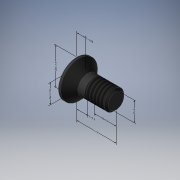
# Autodesk Inventor part: Senkschraube DIN ≈965 M4x8 51305.040.008(High)
Saved by Autodesk Inventor 2019 (Build 230136000, 136)
## iProperties
Created: 2022-09-09
Part Number: Senkschraube DIN ≈965 M4x8 51305.040.008(High)
Material: Generic
Catalog Web Link: www.cadenas.de
Description: DIN ≈965-Counter sunk screws with torx
Vendor: FABORY
Document SubType Name: Modeling
Designer: psAdmin
Manufacturer: FABORY
Mass: 1 g
Surface Area: 2.10234 cm^2
Volume: 0.118629 cm^3
Density: 1 g/cm^3
Appearance: PSOLRGB-175-175-175
Category: PARTsolutions
Company: FABORY
Title: Senkschraube DIN ≈965 M4x8
Author: Cadenas PARTsolutions
Comments: Counter sunk screws with torx
PSOL_IDENT_0: {$CADENAS_DATA/23d-libs/fabory/6_screws/din_965_v2.prj},220 {VTYP=3D},{NB=Senkschraube DIN ≈965 M4x8
PSOL_IDENT_1: 51305.040.008(High)},{LINA=Senkschraube DIN ≈965 M4x8},{NN=DIN ≈965},{DATE=02.05.2022 11:12:59},{GE
PSOL_IDENT_2: OMDATE=13.03.2019 09:47:59},{VERSION=},{LINEID=54070},{WBVAR=LOD},{WBNUMERIC=}  {NB=Senkschraube DIN
PSOL_IDENT_3: ≈965 M4x8 51305.040.008(High)},{LINA=Senkschraube DIN ≈965 M4x8},{KT=DUMMY},{CNSORDERNO=51305.040.0
PSOL_IDENT_4: 08},{NENNID=M4x8},{D=4.000},{L=8},{ERPPDMNUMBER=51305.040.008},{BRAND=Fabory},{STANDARD=DIN ≈965},{T
PSOL_IDENT_5: HREAD=Metric thread},{THREADDIRECTION=},{STYLE=},{TYPE=Machine screw},{GRADE=A2},{BASICMATERIAL=Stai
PSOL_IDENT_6: nless steel},{SURFACETREATMEN=},{HEADSHAPE=Countersunk head},{DRIVINGFEATURE=Hexalobular},{CNSMASSEX
PSOL_IDENT_7: ACT=0.0009},{COLOR=},{COMPARABLESTAND=ISO≈14581;NF≈E25-119-1},{ADDITIONALINFO=Metric},{ROHS=Y},{APPR
PSOL_IDENT_8: OVAL=},{EANCODE=8715494160254},{INTRASTCODE=},{ECLASS=},{UNSPSC=31161504},{ETIM=EC000887},{URL=https
PSOL_IDENT_9: ://www.fabory.com/en-GB/p/51305040008},{PACKAGING=MIN},{VARIANT=MIN},{FABNENN=},{FABGEO=},{FABARTICL
PSOL_IDENT_10: ENR=51305.040.008},{FABNETWEIGHT=0.900},{NENN=M4x8},{D3=3.141},{P=0.700},{DIN962THREAD=},{XLH=0},{DI
PSOL_IDENT_11: N962OPT2=},{OPTIONS2L='',' - ','din_962_std_mid.jpg'},{DIN962OPT3=},{OPTIONSS='',' - ','din_962_std_
PSOL_IDENT_12: gew.jpg'},{B=4.400},{B2=22.000},{A1=1.400},{DK=7.50},{K=2.200},{R=0.400},{X=1.25},{NR=20},{A=3.95},{
PSOL_IDENT_13: T=1.66},{NRP=MIN},{M=MIN},{SCLN=3.5},{SCDN=2.88},{SCLK=2.1},{Z0H=0.8},{Z0D2=8},{Z1H=0.8},{Z1D2=9},{Z
PSOL_IDENT_14: 2H=1},{Z2D2=12},{SD1=1},{SLE=2.2},{FLDP=2.5},{CPDZ=2},{TCDT=0},{SDDP=2.5},{SDZ1=1},{LDDP=2.5},{LDZ2=
PSOL_IDENT_15: 2},{DIN962FTHREAD=0},{VERS=1},{CNSAVOID=0},{DIST=0.31},{LINK1=51305},{LINK2=040},{LINK3=008},{INFOPA
PSOL_IDENT_16: TH=https://www.fabory.com/en-GB/p/51305040008},{LOD=High},{STANDARDSMALL=din_965_v2.png}
NB: Senkschraube DIN ≈965 M4x8 51305.040.008(High)
NN: DIN ≈965
NT: Counter sunk screws with torx
NBSYN: Senkschraube DIN ≈965 $NENN. $CNSORDERNO.($LOD.)
LINA: Senkschraube DIN ≈965 M4x8
CATALOG: Fabory
ROWDESC: M4x8
OFFICIAL_STANDARD_NUMBERS: ISO 14581
CNSORDERNO: 51305.040.008
NENNID: M4x8
D: 4
L: 8
BRAND: Fabory
STANDARD: DIN ≈965
THREAD: Metric thread
TYPE: Machine screw
GRADE: A2
BASICMATERIAL: Stainless steel
HEADSHAPE: Countersunk head
DRIVINGFEATURE: Hexalobular
CNSMASSEXACT: 0.001
COMPARABLESTAND: ISO≈14581;NF≈E25-119-1
ROHS: Y
EANCODE: 8715494160254
UNSPSC: 31161504
ETIM: EC000887
URL: https://www.fabory.com/en-GB/p/51305040008
D3: 3.141
P: 0.7
B: 4.4
B2: 22
A1: 1.4
DK: 7.5
K: 2.2
R: 0.4
X: 1.25
NR: 20
A: 3.95
T: 1.66
NRP: 0
M: 0
SUPPLIER: FABORY
ARTICLENO: Senkschraube DIN ≈965 M4x8 51305.040.008(High)
BOMINFO: Senkschraube DIN ≈965 M4x8
CREATOR: CADENAS GmbH
Autodesk Inventor part; units mm, degrees
sketch "Skizze_5" plane through (0, 0, 0) normal (0, 0, 1) x (1, 0, 0)
  line L0 (8, 0) -> (0, 0)
  line L1 (0, 0) -> (0, 3.75)
  line L2 (0, 3.75) -> (0.45, 3.75)
  line L3 (0.45, 3.75) -> (2.2, 2)
  line L4 (2.2, 2) -> (7.5705, 2)
  line L5 (7.5705, 2) -> (8, 1.5705)
  line L6 (8, 1.5705) -> (8, 0)
  line L7 (8, 0) -> (0, 0)
  constraints: 16 end point
revolve "Revolution1" add sketch "Skizze_5" angle 360 about axis through (8, 0, 0) along (1, 0, 0)
thread "Thread1" size "M4x0.7" class "6g" standard "ISO Metric profile" length 3.9705
sketch "Sketch_1" plane through (0, 0, 0) normal (0, 0, 1) x (1, 0, 0)
  line L0 (1.66, 0) -> (0, 0)
  line L1 (0, 0) -> (0, 1.975)
  line L2 (0, 1.975) -> (1.66, 1.975)
  line L3 (1.66, 1.975) -> (1.66, 0)
  line L4 (1.66, 0) -> (0, 0)
  constraints: 10 end point
revolve "Revolution2" cut sketch "Sketch_1" angle 360 about axis through (1.66, 0, 0) along (1, 0, 0)
sketch "Sketch_2" plane through (0, 0, 0) normal (0, 0, 1) x (1, 0, 0)
  line L0 (2.8003, 0) -> (1.66, 0)
  line L1 (1.66, 0) -> (1.66, 1.975)
  line L2 (1.66, 1.975) -> (2.8003, 0)
  line L3 (2.8003, 0) -> (1.66, 0)
  constraints: 8 end point
revolve "Revolution3" cut sketch "Sketch_2" angle 360 about axis through (2.8003, 0, 0) along (1, 0, 0)
sketch "Sketch_3" plane through (0, 0, 0) normal (1, 0, 0) x (0, 1, 0)
  circle A0 centre (0, 0) radius 2.37
  arc A1 (-0.5027, 1.6394) -> (-1.1684, 1.2551) centre (-0.79, 1.3683) ccw
  arc A2 (-1.6711, 0.3843) -> (-1.1684, 1.2551) centre (-1.8307, 1.0569) ccw
  arc A3 (-1.6711, 0.3843) -> (-1.6711, -0.3843) centre (-1.58, 0) ccw
  arc A4 (-1.1684, -1.2551) -> (-1.6711, -0.3843) centre (-1.8307, -1.0569) ccw
  arc A5 (-1.1684, -1.2551) -> (-0.5027, -1.6394) centre (-0.79, -1.3683) ccw
  arc A6 (0.5027, -1.6394) -> (-0.5027, -1.6394) centre (0, -2.1139) ccw
  arc A7 (0.5027, -1.6394) -> (1.1684, -1.2551) centre (0.79, -1.3683) ccw
  arc A8 (1.6711, -0.3843) -> (1.1684, -1.2551) centre (1.8307, -1.0569) ccw
  arc A9 (1.6711, -0.3843) -> (1.6711, 0.3843) centre (1.58, 0) ccw
  arc A10 (1.1684, 1.2551) -> (1.6711, 0.3843) centre (1.8307, 1.0569) ccw
  arc A11 (1.1684, 1.2551) -> (0.5027, 1.6394) centre (0.79, 1.3683) ccw
  arc A12 (-0.5027, 1.6394) -> (0.5027, 1.6394) centre (0, 2.1139) ccw
  constraints: 24 point on circle, 13 centre point
extrude "Extrusion1" add sketch "Sketch_3" along normal blind 1.66
sketch "Sketch_4" plane through (0, 0, 0) normal (0, 0, 1) x (1, 0, 0)
  line L0 (1.1403, 0) -> (-1.66, 0)
  line L1 (-1.66, 0) -> (-1.66, 1.975)
  line L2 (-1.66, 1.975) -> (0, 1.975)
  line L3 (0, 1.975) -> (1.1403, 0)
  line L4 (1.1403, 0) -> (-1.66, 0)
  constraints: 10 end point
revolve "Revolution4" cut sketch "Sketch_4" angle 360 about axis through (1.1403, 0, 0) along (1, 0, 0)
ref_plane "IP1_XY" through (0, 0, 0) normal (1, 0, 0) x (0, 0, -1)
ref_plane "IP1_YZ" through (0, 0, 0) normal (0, 0, -1) x (0, 1, 0)
ref_plane "IP1_ZX" through (0, 0, 0) normal (0, 1, 0) x (1, 0, 0)
ref_plane "IP2_XY" through (2.2, 0, 0) normal (1, 0, 0) x (0, 0, -1)
ref_plane "IP2_YZ" through (2.2, 0, 0) normal (0, 0, -1) x (0, 1, 0)
ref_plane "IP2_ZX" through (2.2, 0, 0) normal (0, 1, 0) x (1, 0, 0)
ref_plane "IP3_XY" through (8, 0, 0) normal (1, 0, 0) x (0, 0, -1)
ref_plane "IP3_YZ" through (8, 0, 0) normal (0, 0, -1) x (0, 1, 0)
ref_plane "IP3_ZX" through (8, 0, 0) normal (0, 1, 0) x (1, 0, 0)
body "Solid1"
